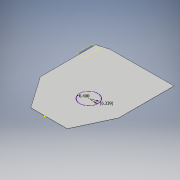
# Autodesk Inventor part: side cover plate.ipt-01
Saved by Autodesk Inventor 2018 (Build 220112000, 112)
## iProperties
Created: 2018-05-29
Part Number: side cover plate.ipt-01
Material: Generic
Document SubType Name: Modeling
Designer: p446024
Density: 1 g/cm^3
Appearance: Default
Author: p446024
Autodesk Inventor part; units mm, degrees
ref_plane "YZ Plane" through (0, 0, 0) normal (1, 0, 0) x (0, 1, 0)
ref_plane "XZ Plane" through (0, 0, 0) normal (0, 1, 0) x (-1, 0, 0)
ref_plane "XY Plane" through (0, 0, 0) normal (0, 0, 1) x (1, 0, 0)
ref_plane "Work Plane1" through (-244.516826, 0, -292.10783) normal (0, -1, 0) x (1, 0, 0)
sketch "Sketch1" plane through (-244.516826, 0, -292.10783) normal (0, -1, 0) x (1, 0, 0)
  line L0 (-82.234926, -443.016385) -> (-82.234926, 4.14342)
  line L1 (16.056549, -523.499895) -> (-89.634926, -493.408338)
  line L2 (-82.234926, 4.14342) -> (116.599095, 288.10783)
  line L3 (116.599095, 288.10783) -> (240.516826, 288.10783)
  line L4 (590.833218, -28.092085) -> (443.497514, 287.870352)
  line L5 (590.833218, -526.137374) -> (590.833218, -28.092085)
  point P0 (244.516826, 292.10783)
  constraints: 7 coincident, 6 end point
sketch "Sketch2" plane through (-244.516826, 0, -292.10783) normal (0, -1, 0) x (1, 0, 0)
  line L0 (16.056549, -523.499895) -> (-82.234926, -495.466532)
  line L1 (-82.234926, -495.466532) -> (-82.234926, 4.14342)
  line L2 (-82.234926, 4.14342) -> (116.599095, 288.10783)
  line L3 (116.599095, 288.10783) -> (443.497514, 287.870352)
  line L4 (443.497514, 287.870352) -> (590.833218, -28.092085)
  line L5 (590.833218, -28.092085) -> (590.833218, -526.137374)
  line L6 (590.833218, -523.499895) -> (16.056549, -523.499895)
  point P0 (244.516826, 292.10783)
  constraints: 14 end point, 1 parallel, 1 perpendicular, 1 vertical
sketch "Sketch2 outline for Plate extrude" plane through (-244.516826, 0, -292.10783) normal (0, -1, 0) x (1, 0, 0)
  line L0 (16.056549, -523.499895) -> (-82.234926, -495.466532)
  line L1 (-82.234926, -495.466532) -> (-82.234926, 4.14342)
  line L2 (-82.234926, 4.14342) -> (116.599095, 288.10783)
  line L3 (116.599095, 288.10783) -> (443.497514, 287.870352)
  line L4 (443.497514, 287.870352) -> (590.833218, -28.092085)
  line L5 (590.833218, -28.092085) -> (590.833218, -526.137374)
  line L6 (590.833218, -526.137374) -> (16.056549, -523.499895)
extrude "Plate extrude" add sketch "Sketch2 outline for Plate extrude" against normal blind 1.6
sketch "Sketch3" plane through (-244.516826, 0, -292.10783) normal (0, -1, 0) x (1, 0, 0)
  circle A0 centre (303.423661, -47.967523) radius 80.5 construction
  circle A1 centre (303.423661, -45.120279) radius 75 construction
  line L0 (153.423661, 104.879721) -> (453.423661, 104.879721)
  line L1 (453.423661, 104.879721) -> (453.423661, -195.120279)
  line L2 (453.423661, -195.120279) -> (153.423661, -195.120279)
  line L3 (153.423661, -195.120279) -> (153.423661, 104.879721)
  line L4 (153.423661, 104.879721) -> (453.423661, -195.120279) construction
  line L5 (453.423661, 104.879721) -> (153.423661, -195.120279) construction
  point P0 (244.516826, 292.10783)
  dimension "d3" = 300
  dimension "d4" = 300
  constraints: 12 end point, 2 midpoint, 2 parallel, 1 horizontal, 1 perpendicular
  measures "d3" distance of L1.end L2.end
  measures "d4" distance of L0.end L1.end
extrude "Tailstock door" [suppressed]
sketch "Sketch4" plane through (-244.516826, 0, -292.10783) normal (0, -1, 0) x (1, 0, 0)
  circle A0 centre (303.423661, -45.120279) radius 75 construction
  circle A1 centre (303.423661, -45.120279) radius 81.28
  circle A2 centre (303.423661, -45.330045) radius 80.5 construction
  point P0 (244.516826, 292.10783)
  dimension "d7" = 162.56
  dimension "d8" = 161
  constraints: 1 centre point, 1 coincident
  measures "d7" diameter of A1
  measures "d8" diameter of A2
extrude "Headstock cut out" [suppressed]
sketch "Sketch5" plane through (-244.516826, 1.6, -292.10783) normal (0, 1, 0) x (1, 0, 0)
  point P0 (244.516826, -292.10783)
  point P1 (303.423661, 45.330045)
body "Solid1"
